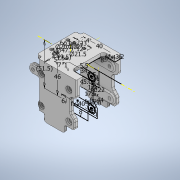
# Autodesk Inventor part: direct drive mount
Saved by Autodesk Inventor 2020.2 (Build 242310000, 310)
## iProperties
Created: 2020-07-21
Part Number: direct drive mount
Material: Generic
Document SubType Name: Modeling
Designer: boxi
Density: 1 g/cm^3
Appearance: Default
Author: boxi
Autodesk Inventor part; units mm, degrees
ref_plane "YZ Plane" through (0, 0, 0) normal (1, 0, 0) x (0, 1, 0)
ref_plane "XZ Plane" through (0, 0, 0) normal (0, 1, 0) x (-1, 0, 0)
ref_plane "XY Plane" through (0, 0, 0) normal (0, 0, 1) x (1, 0, 0)
sketch "Sketch1" plane through (0, 0, 0) normal (0, 1, 0) x (-1, 0, 0)
  line L0 (6, -10.75) -> (-6, -10.75) construction
  circle A0 centre (6, -10.75) radius 1.8 construction
  circle A1 centre (-6, -10.75) radius 1.8 construction
  line L1 (30.5067, 0) -> (-64.0403, 0) projected
  line L2 (0, -36.1225) -> (0, 23.5351) construction
  line L3 (11, 15.0126) -> (11, -15.0126) construction
  line L4 (-29, -23.6) -> (11, -23.6)
  line L5 (11, -23.6) -> (11, 0) construction
  line L6 (5.99, -10.75) -> (6.01, -10.75) construction
  line L7 (5.99, -8.95) -> (6.01, -8.95)
  line L8 (6.01, -12.55) -> (5.99, -12.55)
  arc A2 (5.99, -8.95) -> (5.99, -12.55) centre (5.99, -10.75) ccw
  arc A3 (6.01, -12.55) -> (6.01, -8.95) centre (6.01, -10.75) ccw
  line L9 (-6.01, -10.75) -> (-5.99, -10.75) construction
  line L10 (-6.01, -8.95) -> (-5.99, -8.95)
  line L11 (-5.99, -12.55) -> (-6.01, -12.55)
  arc A4 (-6.01, -8.95) -> (-6.01, -12.55) centre (-6.01, -10.75) ccw
  arc A5 (-5.99, -12.55) -> (-5.99, -8.95) centre (-5.99, -10.75) ccw
  line L12 (11, -23.6) -> (11, -27.6)
  line L13 (11, -27.6) -> (-29, -27.6)
  line L14 (-29, -27.6) -> (-29, -23.6)
  line L15 (11, -23.6) -> (17, -23.6)
  line L16 (17, -23.6) -> (17, 0)
  line L17 (-29, -27.6) -> (-35, -27.6)
  line L18 (-35, -27.6) -> (-35, -19.6)
  line L19 (-29, -23.6) -> (-35, -23.6)
  line L20 (-35, -19.6) -> (-21, -19.6)
  line L21 (-21, -19.6) -> (-21, 0)
  line L22 (-29, -24.4) -> (-35, -24.4)
  circle A6 centre (13.01, -10) radius 1.8 construction
  line L23 (13.11, -10) -> (12.91, -10) construction
  line L24 (13.11, -8.2) -> (12.91, -8.2)
  line L25 (12.91, -11.8) -> (13.11, -11.8)
  arc A7 (13.11, -11.8) -> (13.11, -8.2) centre (13.11, -10) ccw
  arc A8 (12.91, -8.2) -> (12.91, -11.8) centre (12.91, -10) ccw
  point P0 (0, 0)
  dimension "d0" = 3.6
  dimension "d2" = 12
  dimension "d3" = 17
  dimension "d7" = 0.02
  dimension "d8" = 21.5
  dimension "d9" = 40
  dimension "d10" = 47.2
  dimension "d11" = 4
  dimension "d26" = 23
  dimension "d29" = 4
  dimension "d32" = 3.2
  dimension "d33" = 6
  dimension "d37" = 8
  dimension "d77" = 20
  dimension "d78" = 3.6
  dimension "d79" = 7
  dimension "d112" = 0.2
  constraints: 54 end point, 13 tangent, 12 point on circle, 9 centre point, 7 point on line, 6 perpendicular, 5 horizontal, 4 midpoint, 3 equal radius, 3 parallel, 3 vertical, 2 coincident, 2 collinear, 1 symmetric about line, 1 other
  measures "d0" diameter of A0
  measures "d2" distance of L0.start L0.end
  measures "d3" distance from line of L3 L0.end
  measures "d7" distance of L6.start L6.end
  measures "d8" diameter of L0.end L1
  measures "d9" distance of L4.start L4.end
  measures "d10" diameter of L4 L1
  measures "d11" distance between parallel lines of L13 L4
  measures "d26" distance from line of L16 L0.end
  measures "d29" distance between parallel lines of L4 L20
  measures "d32" distance between parallel lines of L17 L22
  measures "d33" distance between parallel lines of L18 L14
  measures "d37" distance between parallel lines of L21 L14
  measures "d77" diameter of A6.centre L1
  measures "d78" diameter of A6
  measures "d79" horizontal distance of L6.end A6.centre
  measures "d112" distance of L23.start L23.end
sketch "Sketch3" plane through (0, 0, 0) normal (0, 0, 1) x (1, 0, 0)
  line L0 (10.5336, -6.6393) -> (50.5336, -6.6393)
  line L1 (50.5336, -6.6393) -> (50.5336, -46.6393)
  line L2 (50.5336, -46.6393) -> (10.5336, -46.6393)
  line L3 (10.5336, -46.6393) -> (10.5336, -6.6393)
  line L4 (48.0336, -9.1393) -> (13.0336, -9.1393) construction
  line L5 (13.0336, -9.1393) -> (13.0336, -44.1393) construction
  line L6 (13.0336, -44.1393) -> (48.0336, -44.1393) construction
  line L7 (48.0336, -44.1393) -> (48.0336, -9.1393) construction
  circle A0 centre (13.0336, -9.1393) radius 1.8166
  circle A1 centre (48.0336, -9.1393) radius 1.6575
  circle A2 centre (13.0336, -44.1393) radius 2.0127
  circle A3 centre (48.0336, -44.1393) radius 1.6922
  dimension "d55" = 40
  dimension "d56" = 40
  dimension "d57" = 35
  constraints: 16 end point, 4 centre point, 4 coincident, 4 parallel, 2 perpendicular, 1 horizontal, 3 other
  measures "d55" distance of L0.start L0.end
  measures "d56" distance of L0.end L1.end
  measures "d57" distance of L4.start L4.end
sketch "Sketch2" plane through (0, 0, 0) normal (0, 0, 1) x (1, 0, 0)
  line L0 (-40.1655, 0) -> (79.9928, 0) projected
  line L1 (0, -71.4) -> (0, 11.9) projected
  circle A0 centre (-8, -10.5) radius 1.75
  circle A1 centre (26, -10.5) radius 1.75
  circle A2 centre (-8, -44.5) radius 1.75
  circle A3 centre (26, -44.5) radius 1.75
  line L2 (-11, 0) -> (29, 0) projected
  line L3 (-11, 0) -> (-11, -51.5)
  line L4 (-11, -51.5) -> (29, -51.5)
  line L5 (-11, -5.5) -> (29, -5.5) construction
  line L6 (-8, -10.5) -> (26, -10.5) construction
  line L7 (26, -10.5) -> (26, -44.5) construction
  line L8 (26, -44.5) -> (-8, -44.5) construction
  line L9 (-8, -44.5) -> (-8, -10.5) construction
  line L10 (-11, -49.5) -> (29, -49.5) construction
  line L11 (9, -5.5) -> (9, -51.5) construction
  line L12 (-11, -27.5) -> (31.8635, -27.5) construction
  line L13 (29, 0) -> (62.8273, 0)
  line L14 (35, -17.5) -> (29.5, -17.5)
  line L15 (27.5, -19.5) -> (27.5, -35)
  line L16 (35, 0) -> (35, -17.5)
  line L17 (33, -51.5) -> (29, -51.5)
  line L18 (33, -40.5) -> (33, -51.5)
  circle A4 centre (26, -10.5) radius 3.75
  circle A5 centre (-8, -10.5) radius 3.75
  circle A6 centre (26, -44.5) radius 3.75
  circle A7 centre (-8, -44.5) radius 3.75
  line L19 (21.5, -49.5) -> (21.5, -59.5)
  line L20 (21.5, -59.5) -> (-5, -59.5)
  line L21 (-5, -59.5) -> (-5, -49.5)
  line L22 (27.5, -35) -> (33, -40.5)
  line L23 (29.5, -17.5) -> (27.5, -19.5)
  line L24 (-11, -6) -> (-23, -6)
  line L25 (-23, -6) -> (-23, -16)
  line L26 (-23, -16) -> (-11, -16)
  circle A8 centre (-18, -11) radius 1.8
  circle A9 centre (-8, -10.5) radius 4.75
  circle A10 centre (-8, -44.5) radius 4.75
  circle A11 centre (26, -10.5) radius 4.75
  circle A12 centre (26, -44.5) radius 4.75
  line L27 (26, -49.25) -> (-8, -49.25)
  line L28 (26, -39.75) -> (-8, -39.75)
  line L29 (26, -5.75) -> (-8, -5.75)
  line L30 (26, -15.25) -> (-8, -15.25)
  point P0 (0, 0)
  point P1 (27.5, -17.5)
  point P2 (47.5, 0)
  point P3 (9, -44.5)
  point P4 (9, -49.5)
  point P5 (21.5, -51.5)
  point P6 (-5, -51.5)
  dimension "d16" = 5.5
  dimension "d17" = 34
  dimension "d18" = 34
  dimension "d19" = 46
  dimension "d20" = 51.5
  dimension "d21" = 44
  dimension "d22" = 22
  dimension "d23" = 3.5
  dimension "d51" = 40
  dimension "d52" = 1.5
  dimension "d54" = 12
  dimension "d58" = 7.5
  dimension "d63" = 7
  dimension "d67" = 8
  dimension "d71" = 6
  dimension "d72" = 6
  dimension "d83" = 17.5
  dimension "d84" = 45
  dimension "d85" = 2
  dimension "d87" = 45
  dimension "d98" = 7
  dimension "d99" = 3.6
  dimension "d100" = 5
  dimension "d101" = 5
  dimension "d102" = 5
  dimension "d103" = 1
  dimension "d110" = 9.5
  dimension "d111" = 11
  constraints: 57 end point, 13 centre point, 12 coincident, 11 point on line, 9 equal radius, 8 point on circle, 7 perpendicular, 7 tangent, 5 horizontal, 4 midpoint, 4 vertical, 3 parallel, 1 vertical alignment, 2 other
  measures "d16" distance between parallel lines of L5 L0
  measures "d17" distance of L6.start L6.end
  measures "d18" distance of L6.end L7.end
  measures "d19" distance between parallel lines of L4 L5
  measures "d20" distance between parallel lines of L4 L0
  measures "d21" distance between parallel lines of L10 L5
  measures "d22" distance between parallel lines of L12 L5
  measures "d23" diameter of A0
  measures "d51" distance of L10.start L10.end
  measures "d52" distance between parallel lines of L7 L15
  measures "d54" distance between parallel lines of L14 L5
  measures "d58" diameter of A4
  measures "d63" distance between parallel lines of L18 L7
  measures "d67" distance between parallel lines of L4 L20
  measures "d71" distance between parallel lines of L3 L21
  measures "d72" distance between parallel lines of L15 L19
  measures "d83" distance of point (27.5, -17.5) L15.end
  measures "d84" angle of L15 L22
  measures "d85" distance of L14.end point (27.5, -17.5)
  measures "d87" angle of L14 L23
  measures "d98" distance from line of L3 A8.centre
  measures "d99" diameter of A8
  measures "d100" distance from line of L24 A8.centre
  measures "d101" distance from line of L26 A8.centre
  measures "d102" distance from line of L25 A8.centre
  measures "d103" radial gap between concentric circles of A5 A9
  measures "d110" diameter of A9
  measures "d111" distance from line of A8.centre L0
extrude "Extrusion1" add sketch "Sketch1" along normal blind 4
extrude "Extrusion5" add sketch "Sketch2" along normal blind 4 from surface at -27.6 contours L0 L16 L14 L23 L15 L22 L18 L17 L4 L1 L27 A12 L28 L30 A11 L29 | L1 L29 A9 L3 L0 | L29 A11 L30 L1 | L1 L30 A9 L29 | L3 A9 L26 L25 L24 | L1 L28 A10 L3 A9 L30 | A11 | A9 L3 A5 | L3 A5 A9 | L28 A12 L27 L1 | L1 L27 A10 L28 | A5 L3 | L3 A5 | L1 L4 L3 A10 L27 | A12 | A10 L3 A7 | A7 L3 | A4 | A6 picked at (-10.4804, -40.8767) picked at (-10.5833, -44.5)
extrude "Extrusion7" add sketch "Sketch2" along normal blind 2.4 from surface at -27.6 contours L4 L19 L20 L1 | L1 L20 L21 L4
chamfer "Chamfer4" distance 4.5 angle 45 1 edges at (12, 0, -23.6)
extrude "Extrusion8" add sketch "Sketch2" along normal blind 5.5 from surface at -27.6 contours L29 A11 L30 L1 | L1 L30 A9 L29 | A11 | A9 L3 A5 | L3 A5 A9 | L28 A12 L27 L1 | L1 L27 A10 L28 | A5 L3 | L3 A5 | A12 | A10 L3 A7 | L3 A7 A10 | A7 L3 | L3 A7 | A4 | A6
extrude "Extrusion6" cut sketch "Sketch2" along normal blind 2.8 from surface at -27.6 contours A5 L3 | L3 A5 | A7 L3 | L3 A7 | A0 | A1 | A2 | A3 | A4 | A6
fillet "Fillet3" radius 1 24 edges at (-17, 0, -11.8) (-11, -1, -27.6) (27.5, -27.25, -27.6) (35, -6.75, -27.6) (32.25, -17.5, -27.6) (33, -46, -27.6) (-5, -55.5, -25.2) (21.5, -55.5, -25.2) (8.25, -51.5, -25.2) (-5, -51.5, -26.4) (21.5, -51.5, -26.4) (-5, -55.5, -27.6) (21.5, -55.5, -27.6) (-11, -51.5, -25.6) (27.25, -51.5, -27.6) (-8, -51.5, -27.6) (28.5, -18.5, -27.6) (30.25, -37.75, -27.6) (-17, -6, -27.6) (-23, -11, -27.6) (-17, -16, -27.6) (-11, -28.4086, -27.6) (-11, -49.8414, -27.6) (-12.75, -44.5, -27.6)
fillet "Fillet3" radius 4 9 edges at (21, 1.75, -19.6) (-23, -16, -25.6) (-23, -6, -25.6) (35, -17.5, -25.6) (27.5, -35, -25.6) (33, -40.5, -25.6) (33, -51.5, -25.6) (21.5, -59.5, -26.4) (-5, -59.5, -26.4)
fillet "Fillet3" radius 2 8 edges at (-11, 2, -23.6) (-17, 2, -23.6) (29.5, -17.5, -25.6) (27.5, -19.5, -25.6) (-11, -16, -25.6) (-11, -40.8173, -25.6) (-11, -48.1827, -25.6) (-11, -6, -25.6)
chamfer "Chamfer7" distance 1.5 angle 45 11 edges at (30.75, -44.5, -23.6) (9, -49.25, -23.6) (-9.5921, -48.9752, -23.6) (-11.2685, -47.9466, -23.6) (9, -39.75, -23.6) (-11.2685, -41.0534, -23.6) (-9.5921, -40.0248, -23.6) (-12.75, -10.5, -23.6) (9, -5.75, -23.6) (30.75, -10.5, -23.6) (9, -15.25, -23.6)
chamfer "Chamfer6" distance 1 angle 45 4 edges at (-11.75, -44.5, -24.8) (-11.75, -10.5, -24.8) (22.25, -10.5, -24.8) (22.25, -44.5, -24.8)
mirror "Mirror1" about plane through (0, 0, 0) normal (0, 0, 1)
equation "\"d32\" = 0.8 * d11"
equation "\"d21\" = extruder_length"
equation "\"d22\" = 0.5 * extruder_length"
equation "\"extruder_length\" = 44"
body "Solid1"
